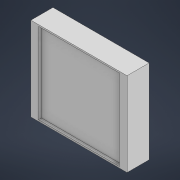
# Autodesk Inventor part: End-Effector
Saved by Autodesk Inventor 2022 (Build 260153000, 153)
## iProperties
Created: 2023-04-20
Part Number: End-Effector
Material: Generic
Document SubType Name: Modeling
Designer: Karl
Density: 1 g/cm^3
Appearance: Default
Author: Karl
Autodesk Inventor part; units mm, degrees
ref_plane "YZ Plane" through (0, 0, 0) normal (1, 0, 0) x (0, 1, 0)
ref_plane "XZ Plane" through (0, 0, 0) normal (0, 1, 0) x (-1, 0, 0)
ref_plane "XY Plane" through (0, 0, 0) normal (0, 0, 1) x (1, 0, 0)
sketch "Sketch3" plane through (0, 0, 0) normal (0, 0, 1) x (1, 0, 0)
  line L0 (0, 0) -> (-55.38, 0)
  line L1 (-55.38, 0) -> (-55.38, 47.03)
  line L2 (-55.38, 47.03) -> (0, 47.03)
  line L3 (0, 47.03) -> (0, 0)
  line L4 (5, -5) -> (5, 52.03)
  line L5 (5, 52.03) -> (-60.38, 52.03)
  line L6 (5, -5) -> (-60.38, -5)
  line L7 (-60.38, -5) -> (-60.38, 52.03)
  dimension "d26" = 47.03
  dimension "d27" = 55.38
  constraints: 16 end point, 3 perpendicular, 2 horizontal, 2 parallel, 1 vertical
  measures "d26" distance of L2.end L0.start
  measures "d27" distance of L0.start L0.end
extrude "Extrusion10" add sketch "Sketch3" along normal blind 10
sketch "Sketch10" plane through (0, 0, 10) normal (0, 0, 1) x (1, 0, 0)
  line L0 (-60.38, 52.03) -> (5, 52.03)
  line L1 (5, 52.03) -> (5, -5)
  line L2 (5, -5) -> (-60.38, -5)
  line L3 (-60.38, -5) -> (-60.38, 52.03)
  point P0 (0, 0)
  constraints: 8 end point, 2 parallel, 1 horizontal, 1 perpendicular
extrude "Extrusion11" add sketch "Sketch10" along normal blind 5
sketch "Sketch11" plane through (0, 0, 15) normal (0, 0, 1) x (1, 0, 0)
  line L0 (5, -5) -> (-0.19, -5)
  line L1 (-0.19, -5) -> (-0.19, -3.985)
  line L2 (-0.19, -5) -> (0.825, -5) construction
  line L3 (-0.19, -3.985) -> (-55.19, -3.985)
  line L4 (-55.19, -3.985) -> (-55.19, 51.015)
  line L5 (-55.19, 51.015) -> (-0.19, 51.015)
  line L6 (-0.19, 51.015) -> (-0.19, -3.985)
  point P0 (0, 0)
  point P1 (-60.38, -5)
  point P2 (-60.38, 52.03)
  dimension "d73" = 65.38
  dimension "d76" = 5.19
  dimension "d78" = 1.015
  dimension "d79" = 90
  dimension "d80" = 55
  dimension "d81" = 55
  constraints: 14 end point, 2 horizontal, 2 parallel, 2 perpendicular
  measures "d73" distance of point (-60.38, -5) L0.start
  measures "d76" distance of L0.start L0.end
  measures "d78" distance of L0.end L1.end
  measures "d79" angle of L2 L1
  measures "d80" distance of L4.end L5.end
  measures "d81" distance of L3.end L4.end
extrude "Extrusion12" cut sketch "Sketch11" against normal blind 2
body "Solid3"
